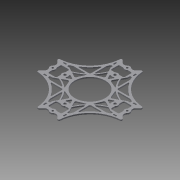
# Autodesk Inventor part: Middle Plate Under
Saved by Autodesk Inventor 2014 SP1 (Build 180222100, 222)
## iProperties
Created: 2014-07-28
Part Number: Middle Plate Under
Material: Generic
Document SubType Name: Modeling
Designer: Ryan
Density: 1 g/cm^3
Appearance: Default
Author: Ryan
Autodesk Inventor part; units mm, degrees
(part 1 of 2)
ref_plane "YZ Plane" through (0, 0, 0) normal (1, 0, 0) x (0, 1, 0)
ref_plane "XZ Plane" through (0, 0, 0) normal (0, 1, 0) x (-1, 0, 0)
ref_plane "XY Plane" through (0, 0, 0) normal (0, 0, 1) x (1, 0, 0)
sketch "Middle Plate Under" plane through (0, 0, 0) normal (0, 0, 1) x (1, 0, 0)
  arc A0 (50.1297, 0.9388) -> (0.939, 50.1217) centre (-2.2631, -2.2716) ccw
  arc A1 (50.1297, 0.9388) -> (51.1278, 0) centre (51.1278, 1) ccw
  arc A2 (0, 51.1198) -> (0.939, 50.1217) centre (1, 51.1198) ccw
  line L0 (5.9986, 74.9303) -> (5.9986, 74.6246)
  arc A3 (5.9986, 74.9303) -> (4.5341, 78.4659) centre (0.9986, 74.9303) ccw
  arc A4 (0.9376, 85.8703) -> (50.1218, 135.0623) centre (-2.3433, 138.3348) ccw
  arc A5 (0.9376, 85.8703) -> (0, 84.8722) centre (1, 84.8722) ccw
  arc A6 (51.1198, 136) -> (50.1218, 135.0623) centre (51.1198, 135) ccw
  arc A7 (135.0596, 50.1296) -> (85.8784, 0.9406) centre (138.1819, -2.1735) ccw
  arc A8 (84.8801, 0) -> (85.8784, 0.9406) centre (84.8801, 1) ccw
  arc A9 (135.0596, 50.1296) -> (136, 51.1278) centre (135, 51.1278) ccw
  arc A10 (85.8703, 135.0624) -> (135.0622, 85.8782) centre (138.334, 138.3425) ccw
  arc A11 (85.8703, 135.0624) -> (84.8722, 136) centre (84.8722, 135) ccw
  arc A12 (136, 84.8802) -> (135.0622, 85.8782) centre (135, 84.8802) ccw
  circle A13 centre (27.5084, 68) radius 2.1
  circle A14 centre (108.4916, 68) radius 2.1
  circle A15 centre (68, 108.4916) radius 2.1
  circle A16 centre (68, 27.5084) radius 2.1
  line L1 (14, 83) -> (9, 83)
  line L2 (14, 53) -> (9, 53)
  line L3 (9, 83) -> (9, 85.1)
  line L4 (9, 85.1) -> (14, 85.1)
  line L5 (14, 85.1) -> (14, 83)
  line L6 (14, 53) -> (14, 50.9)
  line L7 (14, 50.9) -> (9, 50.9)
  line L8 (9, 50.9) -> (9, 53)
  line L9 (122, 83) -> (127, 83)
  line L10 (122, 53) -> (127, 53)
  line L11 (127, 83) -> (127, 85.1)
  line L12 (127, 85.1) -> (122, 85.1)
  line L13 (122, 85.1) -> (122, 83)
  line L14 (122, 53) -> (122, 50.9)
  line L15 (122, 50.9) -> (127, 50.9)
  line L16 (127, 50.9) -> (127, 53)
  line L17 (53, 122) -> (53, 127)
  line L18 (83, 122) -> (83, 127)
  line L19 (53, 127) -> (50.9, 127)
  line L20 (50.9, 127) -> (50.9, 122)
  line L21 (50.9, 122) -> (53, 122)
  line L22 (83, 122) -> (85.1, 122)
  line L23 (85.1, 122) -> (85.1, 127)
  line L24 (85.1, 127) -> (83, 127)
  line L25 (53, 14) -> (53, 9)
  line L26 (83, 14) -> (83, 9)
  line L27 (53, 9) -> (50.9, 9)
  line L28 (50.9, 9) -> (50.9, 14)
  line L29 (50.9, 14) -> (53, 14)
  line L30 (83, 14) -> (85.1, 14)
  line L31 (85.1, 14) -> (85.1, 9)
  line L32 (85.1, 9) -> (83, 9)
  line L33 (12.5486, 78.8671) -> (22.185, 78.8671)
  arc A17 (12.5486, 78.8671) -> (10.6486, 76.9671) centre (12.5486, 76.9671) ccw
  line L34 (10.6486, 76.9671) -> (10.6486, 71.42)
  line L35 (24.085, 71.42) -> (24.085, 76.9671)
  arc A18 (24.085, 76.9671) -> (22.185, 78.8671) centre (22.185, 76.9671) ccw
  line L36 (12.5486, 57.1329) -> (22.185, 57.1329)
  arc A19 (10.6486, 59.0329) -> (12.5486, 57.1329) centre (12.5486, 59.0329) ccw
  line L37 (10.6486, 59.0329) -> (10.6486, 64.58)
  line L38 (24.085, 64.58) -> (24.085, 59.0329)
  arc A20 (22.185, 57.1329) -> (24.085, 59.0329) centre (22.185, 59.0329) ccw
  arc A21 (10.6486, 64.58) -> (10.6486, 71.42) centre (7.1826, 68) ccw
  arc A22 (24.085, 71.42) -> (24.085, 64.58) centre (27.505, 68) ccw
  line L39 (123.4514, 78.8671) -> (113.815, 78.8671)
  arc A23 (125.3514, 76.9671) -> (123.4514, 78.8671) centre (123.4514, 76.9671) ccw
  line L40 (125.3514, 76.9671) -> (125.3514, 71.42)
  line L41 (111.915, 71.42) -> (111.915, 76.9671)
  arc A24 (113.815, 78.8671) -> (111.915, 76.9671) centre (113.815, 76.9671) ccw
  line L42 (123.4514, 57.1329) -> (113.815, 57.1329)
  arc A25 (123.4514, 57.1329) -> (125.3514, 59.0329) centre (123.4514, 59.0329) ccw
  line L43 (125.3514, 59.0329) -> (125.3514, 64.58)
  line L44 (111.915, 64.58) -> (111.915, 59.0329)
  arc A26 (111.915, 59.0329) -> (113.815, 57.1329) centre (113.815, 59.0329) ccw
  arc A27 (125.3514, 71.42) -> (125.3514, 64.58) centre (128.8174, 68) ccw
  arc A28 (111.915, 64.58) -> (111.915, 71.42) centre (108.495, 68) ccw
  line L45 (57.1329, 123.4514) -> (57.1329, 113.815)
  arc A29 (59.0329, 125.3514) -> (57.1329, 123.4514) centre (59.0329, 123.4514) ccw
  line L46 (59.0329, 125.3514) -> (64.58, 125.3514)
  line L47 (64.58, 111.915) -> (59.0329, 111.915)
  arc A30 (57.1329, 113.815) -> (59.0329, 111.915) centre (59.0329, 113.815) ccw
  line L48 (78.8671, 123.4514) -> (78.8671, 113.815)
  arc A31 (78.8671, 123.4514) -> (76.9671, 125.3514) centre (76.9671, 123.4514) ccw
  line L49 (76.9671, 125.3514) -> (71.42, 125.3514)
  line L50 (71.42, 111.915) -> (76.9671, 111.915)
  arc A32 (76.9671, 111.915) -> (78.8671, 113.815) centre (76.9671, 113.815) ccw
  arc A33 (64.58, 125.3514) -> (71.42, 125.3514) centre (68, 128.8174) ccw
  arc A34 (71.42, 111.915) -> (64.58, 111.915) centre (68, 108.495) ccw
  line L51 (57.1329, 12.5486) -> (57.1329, 22.185)
  arc A35 (57.1329, 12.5486) -> (59.0329, 10.6486) centre (59.0329, 12.5486) ccw
  line L52 (59.0329, 10.6486) -> (64.58, 10.6486)
  line L53 (64.58, 24.085) -> (59.0329, 24.085)
  arc A36 (59.0329, 24.085) -> (57.1329, 22.185) centre (59.0329, 22.185) ccw
  line L54 (78.8671, 12.5486) -> (78.8671, 22.185)
  arc A37 (76.9671, 10.6486) -> (78.8671, 12.5486) centre (76.9671, 12.5486) ccw
  line L55 (76.9671, 10.6486) -> (71.42, 10.6486)
  line L56 (71.42, 24.085) -> (76.9671, 24.085)
  arc A38 (78.8671, 22.185) -> (76.9671, 24.085) centre (76.9671, 22.185) ccw
  arc A39 (71.42, 10.6486) -> (64.58, 10.6486) centre (68, 7.1826) ccw
  arc A40 (64.58, 24.085) -> (71.42, 24.085) centre (68, 27.505) ccw
  arc A41 (27.6448, 91.2527) -> (44.7476, 108.3555) centre (-2.445, 138.4453) ccw
  arc A42 (27.6448, 91.2527) -> (28.102, 89.6852) centre (28.102, 90.5356) ccw
  arc A43 (46.3151, 107.8983) -> (44.7476, 108.3555) centre (45.4647, 107.8983) ccw
  line L57 (40.2804, 87.1341) -> (22.5335, 87.1334)
  line L58 (44.1891, 89.6852) -> (28.102, 89.6852)
  line L59 (46.3151, 91.8112) -> (46.3151, 107.8983)
  arc A44 (44.1891, 89.6852) -> (46.3151, 91.8112) centre (44.1891, 91.8112) ccw
  arc A45 (27.1963, 78.4533) -> (28.6868, 78.3895) centre (28.007, 79.9485) ccw
  arc A46 (28.6868, 78.3895) -> (40.8045, 85.614) centre (6.3199, 129.6804) ccw
  line L60 (21.3459, 81.6253) -> (27.1963, 78.4533)
  line L61 (30.5408, 76.64) -> (37.2048, 73.0269)
  arc A47 (40.8045, 85.614) -> (40.2804, 87.1341) centre (40.2804, 86.2837) ccw
  arc A48 (91.2524, 108.3555) -> (108.3552, 91.2527) centre (138.445, 138.4453) ccw
  arc A49 (107.898, 89.6852) -> (108.3552, 91.2527) centre (107.898, 90.5356) ccw
  arc A50 (91.2524, 108.3555) -> (89.6849, 107.8983) centre (90.5353, 107.8983) ccw
  line L62 (91.8109, 89.6852) -> (107.898, 89.6852)
  line L63 (89.6849, 91.8112) -> (89.6849, 107.8983)
  arc A51 (89.6849, 91.8112) -> (91.8109, 89.6852) centre (91.8109, 91.8112) ccw
  arc A52 (108.3552, 44.7479) -> (91.2524, 27.6451) centre (138.445, -2.4447) ccw
  arc A53 (108.3552, 44.7479) -> (107.898, 46.3154) centre (107.898, 45.465) ccw
  arc A54 (89.6849, 28.1023) -> (91.2524, 27.6451) centre (90.5353, 28.1023) ccw
  line L64 (91.8109, 46.3154) -> (107.898, 46.3154)
  line L65 (89.6849, 44.1894) -> (89.6849, 28.1023)
  arc A55 (91.8109, 46.3154) -> (89.6849, 44.1894) centre (91.8109, 44.1894) ccw
  arc A56 (30.5752, 77.4043) -> (44.1261, 85.6969) centre (8.4389, 128.7951) ccw
  arc A57 (44.7901, 85.2067) -> (44.1261, 85.6969) centre (44.3973, 85.3694) ccw
  arc A58 (30.5752, 77.4043) -> (30.5408, 76.64) centre (30.7434, 77.0138) ccw
  line L66 (44.7901, 85.2067) -> (40.1822, 74.0823)
  arc A59 (37.2048, 73.0269) -> (40.1822, 74.0823) centre (38.2181, 74.8959) ccw
  line L67 (30.5408, 59.3606) -> (37.2048, 62.9737)
  arc A60 (40.1822, 61.9183) -> (37.2048, 62.9737) centre (38.2181, 61.1047) ccw
  arc A61 (44.1261, 50.3037) -> (30.5752, 58.5963) centre (8.4389, 7.2055) ccw
  arc A62 (44.1261, 50.3037) -> (44.7901, 50.7939) centre (44.3973, 50.6312) ccw
  arc A63 (30.5408, 59.3606) -> (30.5752, 58.5963) centre (30.7434, 58.9868) ccw
  line L68 (44.7901, 50.7939) -> (40.1822, 61.9183)
  line L69 (105.4592, 76.64) -> (98.7952, 73.0269)
  arc A64 (91.8739, 85.6969) -> (105.4248, 77.4043) centre (127.5611, 128.7951) ccw
  arc A65 (91.8739, 85.6969) -> (91.2099, 85.2067) centre (91.6027, 85.3694) ccw
  arc A66 (105.4592, 76.64) -> (105.4248, 77.4043) centre (105.2566, 77.0138) ccw
  line L70 (91.2099, 85.2067) -> (95.8178, 74.0823)
  arc A67 (95.8178, 74.0823) -> (98.7952, 73.0269) centre (97.7819, 74.8959) ccw
  line L71 (105.4592, 59.3606) -> (98.7952, 62.9737)
  arc A68 (98.7952, 62.9737) -> (95.8178, 61.9183) centre (97.7819, 61.1047) ccw
  arc A69 (105.4248, 58.5963) -> (91.8739, 50.3037) centre (127.5611, 7.2055) ccw
  arc A70 (91.2099, 50.7939) -> (91.8739, 50.3037) centre (91.6027, 50.6312) ccw
  arc A71 (105.4248, 58.5963) -> (105.4592, 59.3606) centre (105.2566, 58.9868) ccw
  line L72 (91.2099, 50.7939) -> (95.8178, 61.9183)
  line L73 (59.3603, 105.4595) -> (62.9734, 98.7955)
  arc A72 (61.918, 95.8181) -> (62.9734, 98.7955) centre (61.1044, 97.7822) ccw
  arc A73 (50.3034, 91.8742) -> (58.596, 105.4251) centre (7.2052, 127.5614) ccw
  arc A74 (50.3034, 91.8742) -> (50.7936, 91.2102) centre (50.6309, 91.603) ccw
  arc A75 (59.3603, 105.4595) -> (58.596, 105.4251) centre (58.9865, 105.2569) ccw
  line L74 (50.7936, 91.2102) -> (61.918, 95.8181)
  line L75 (76.6397, 105.4595) -> (73.0266, 98.7955)
  arc A76 (73.0266, 98.7955) -> (74.082, 95.8181) centre (74.8956, 97.7822) ccw
  arc A77 (77.404, 105.4251) -> (85.6966, 91.8742) centre (128.7948, 127.5614) ccw
  arc A78 (85.2064, 91.2102) -> (85.6966, 91.8742) centre (85.3691, 91.603) ccw
  arc A79 (77.404, 105.4251) -> (76.6397, 105.4595) centre (77.0135, 105.2569) ccw
  line L76 (85.2064, 91.2102) -> (74.082, 95.8181)
  line L77 (59.3603, 30.5411) -> (62.9734, 37.2051)
  arc A80 (62.9734, 37.2051) -> (61.918, 40.1825) centre (61.1044, 38.2184) ccw
  arc A81 (58.596, 30.5755) -> (50.3034, 44.1264) centre (7.2052, 8.4392) ccw
  arc A82 (50.7936, 44.7904) -> (50.3034, 44.1264) centre (50.6309, 44.3976) ccw
  arc A83 (58.596, 30.5755) -> (59.3603, 30.5411) centre (58.9865, 30.7437) ccw
  line L78 (50.7936, 44.7904) -> (61.918, 40.1825)
  line L79 (76.6397, 30.5411) -> (73.0266, 37.2051)
  arc A84 (85.6966, 44.1264) -> (77.404, 30.5755) centre (128.7948, 8.4392) ccw
  arc A85 (85.6966, 44.1264) -> (85.2064, 44.7904) centre (85.3691, 44.3976) ccw
  arc A86 (76.6397, 30.5411) -> (77.404, 30.5755) centre (77.0135, 30.7437) ccw
  line L80 (85.2064, 44.7904) -> (74.082, 40.1825)
  arc A87 (74.082, 40.1825) -> (73.0266, 37.2051) centre (74.8956, 38.2184) ccw
  circle A88 centre (68, 68) radius 24.5933
  arc A89 (44.7476, 27.6451) -> (27.6448, 44.7479) centre (-2.445, -2.4447) ccw
  arc A90 (44.7476, 27.6451) -> (46.3151, 28.1023) centre (45.4647, 28.1023) ccw
  arc A91 (28.102, 46.3154) -> (27.6448, 44.7479) centre (28.102, 45.465) ccw
  line L81 (46.3151, 44.1894) -> (46.3151, 28.1023)
  line L82 (44.1891, 46.3154) -> (28.102, 46.3154)
  arc A92 (46.3151, 44.1894) -> (44.1891, 46.3154) centre (44.1891, 44.1894) ccw
  line L83 (64.2924, 102.9057) -> (67.1209, 97.6888)
  arc A93 (67.1209, 97.6888) -> (68.8791, 97.6888) centre (68, 98.1654) ccw
  line L84 (71.7076, 102.9057) -> (68.8791, 97.6888)
  arc A94 (65.6558, 104.2572) -> (70.3442, 104.2572) centre (68, 108.4916) ccw
  arc A95 (65.6558, 104.2572) -> (64.2924, 102.9057) centre (65.1715, 103.3823) ccw
  arc A96 (71.7076, 102.9057) -> (70.3442, 104.2572) centre (70.8285, 103.3823) ccw
  line L85 (64.2924, 33.0943) -> (67.1209, 38.3112)
  arc A97 (68.8791, 38.3112) -> (67.1209, 38.3112) centre (68, 37.8346) ccw
  line L86 (71.7076, 33.0943) -> (68.8791, 38.3112)
  arc A98 (70.3442, 31.7428) -> (65.6558, 31.7428) centre (68, 27.5084) ccw
  arc A99 (64.2924, 33.0943) -> (65.6558, 31.7428) centre (65.1715, 32.6177) ccw
  arc A100 (70.3442, 31.7428) -> (71.7076, 33.0943) centre (70.8285, 32.6177) ccw
  line L87 (33.0946, 71.7079) -> (38.3115, 68.8794)
  arc A101 (38.3115, 67.1212) -> (38.3115, 68.8794) centre (37.8349, 68.0003) ccw
  line L88 (33.0946, 64.2927) -> (38.3115, 67.1212)
  arc A102 (31.7431, 65.6561) -> (31.7431, 70.3445) centre (27.5087, 68.0003) ccw
  arc A103 (33.0946, 71.7079) -> (31.7431, 70.3445) centre (32.618, 70.8288) ccw
  arc A104 (31.7431, 65.6561) -> (33.0946, 64.2927) centre (32.618, 65.1718) ccw
  line L89 (102.906, 71.7079) -> (97.6891, 68.8794)
  arc A105 (97.6891, 68.8794) -> (97.6891, 67.1212) centre (98.1657, 68.0003) ccw
  line L90 (102.906, 64.2927) -> (97.6891, 67.1212)
  arc A106 (104.2575, 70.3445) -> (104.2575, 65.6561) centre (108.4919, 68.0003) ccw
  arc A107 (104.2575, 70.3445) -> (102.906, 71.7079) centre (103.3826, 70.8288) ccw
  arc A108 (102.906, 64.2927) -> (104.2575, 65.6561) centre (103.3826, 65.1718) ccw
  circle A109 centre (7.7484, 68) radius 1.6
  circle A110 centre (128.2516, 68) radius 1.6
  circle A111 centre (68, 128.2516) radius 1.6
  circle A112 centre (68, 7.7484) radius 1.6
  arc A113 (4.7048, 71.2684) -> (4.7048, 64.7316) centre (8.3141, 68) ccw
  arc A114 (5.9986, 61.3754) -> (4.7048, 64.7316) centre (0.9986, 61.3754) ccw
  arc A115 (4.7048, 71.2684) -> (5.9986, 74.6246) centre (0.9986, 74.6246) ccw
  arc A116 (131.2952, 64.7316) -> (131.2952, 71.2684) centre (127.6859, 68) ccw
  arc A117 (131.2952, 64.7316) -> (130.0014, 61.3754) centre (135.0014, 61.3754) ccw
  arc A118 (130.0014, 74.6246) -> (131.2952, 71.2684) centre (135.0014, 74.6246) ccw
  arc A119 (71.2684, 131.2952) -> (64.7316, 131.2952) centre (68, 127.6859) ccw
  arc A120 (71.2684, 131.2952) -> (74.6246, 130.0014) centre (74.6246, 135.0014) ccw
  arc A121 (61.3754, 130.0014) -> (64.7316, 131.2952) centre (61.3754, 135.0014) ccw
  arc A122 (64.7316, 4.7048) -> (71.2684, 4.7048) centre (68, 8.3141) ccw
  arc A123 (64.7316, 4.7048) -> (61.3754, 5.9986) centre (61.3754, 0.9986) ccw
  arc A124 (74.6246, 5.9986) -> (71.2684, 4.7048) centre (74.6246, 0.9986) ccw
  line L91 (17, 83.6623) -> (17, 82.8671)
  arc A125 (18.2965, 85.5345) -> (21.7007, 86.9517) centre (-0.1983, 134.7566) ccw
  arc A126 (18.2965, 85.5345) -> (17, 83.6623) centre (19, 83.6623) ccw
  arc A127 (22.5335, 87.1334) -> (21.7007, 86.9517) centre (22.5336, 85.1334) ccw
  line L92 (18, 81.8671) -> (20.3926, 81.8671)
  arc A128 (17, 82.8671) -> (18, 81.8671) centre (18, 82.8671) ccw
  arc A129 (21.3459, 81.6253) -> (20.3926, 81.8671) centre (20.3926, 79.8671) ccw
  line L93 (40.2804, 48.8659) -> (22.5335, 48.8666)
  arc A130 (28.6868, 57.6105) -> (27.1963, 57.5467) centre (28.007, 56.0515) ccw
  arc A131 (40.8045, 50.386) -> (28.6868, 57.6105) centre (6.3199, 6.3196) ccw
  line L94 (21.3459, 54.3747) -> (27.1963, 57.5467)
  arc A132 (40.2804, 48.8659) -> (40.8045, 50.386) centre (40.2804, 49.7163) ccw
  line L95 (17, 52.3377) -> (17, 53.1329)
  arc A133 (21.7007, 49.0483) -> (18.2965, 50.4655) centre (-0.1983, 1.2434) ccw
  arc A134 (17, 52.3377) -> (18.2965, 50.4655) centre (19, 52.3377) ccw
  arc A135 (21.7007, 49.0483) -> (22.5335, 48.8666) centre (22.5336, 50.8666) ccw
  line L96 (18, 54.1329) -> (20.3926, 54.1329)
  arc A136 (18, 54.1329) -> (17, 53.1329) centre (18, 53.1329) ccw
  arc A137 (20.3926, 54.1329) -> (21.3459, 54.3747) centre (20.3926, 56.1329) ccw
  line L97 (95.7196, 87.1341) -> (113.4665, 87.1334)
  arc A138 (107.3132, 78.3895) -> (108.8037, 78.4533) centre (107.993, 79.9485) ccw
  arc A139 (95.1955, 85.614) -> (107.3132, 78.3895) centre (129.6801, 129.6804) ccw
  line L98 (114.6541, 81.6253) -> (108.8037, 78.4533)
  arc A140 (95.7196, 87.1341) -> (95.1955, 85.614) centre (95.7196, 86.2837) ccw
  line L99 (119, 83.6623) -> (119, 82.8671)
  arc A141 (114.2993, 86.9517) -> (117.7035, 85.5345) centre (136.1983, 134.7566) ccw
  arc A142 (119, 83.6623) -> (117.7035, 85.5345) centre (117, 83.6623) ccw
  arc A143 (114.2993, 86.9517) -> (113.4665, 87.1334) centre (113.4664, 85.1334) ccw
  line L100 (118, 81.8671) -> (115.6074, 81.8671)
  arc A144 (118, 81.8671) -> (119, 82.8671) centre (118, 82.8671) ccw
  arc A145 (115.6074, 81.8671) -> (114.6541, 81.6253) centre (115.6074, 79.8671) ccw
  line L101 (95.7196, 48.8659) -> (113.4665, 48.8666)
  arc A146 (108.8037, 57.5467) -> (107.3132, 57.6105) centre (107.993, 56.0515) ccw
  arc A147 (107.3132, 57.6105) -> (95.1955, 50.386) centre (129.6801, 6.3196) ccw
  line L102 (114.6541, 54.3747) -> (108.8037, 57.5467)
  arc A148 (95.1955, 50.386) -> (95.7196, 48.8659) centre (95.7196, 49.7163) ccw
  line L103 (119, 52.3377) -> (119, 53.1329)
  arc A149 (117.7035, 50.4655) -> (114.2993, 49.0483) centre (136.1983, 1.2434) ccw
  arc A150 (117.7035, 50.4655) -> (119, 52.3377) centre (117, 52.3377) ccw
  arc A151 (113.4665, 48.8666) -> (114.2993, 49.0483) centre (113.4664, 50.8666) ccw
  line L104 (118, 54.1329) -> (115.6074, 54.1329)
  arc A152 (119, 53.1329) -> (118, 54.1329) centre (118, 53.1329) ccw
  arc A153 (114.6541, 54.3747) -> (115.6074, 54.1329) centre (115.6074, 56.1329) ccw
  line L105 (48.8662, 40.2807) -> (48.8669, 22.5339)
  arc A154 (57.547, 27.1966) -> (57.6108, 28.6871) centre (56.0518, 28.0073) ccw
  arc A155 (57.6108, 28.6871) -> (50.3863, 40.8048) centre (6.3199, 6.3202) ccw
  line L106 (54.375, 21.3462) -> (57.547, 27.1966)
  arc A156 (50.3863, 40.8048) -> (48.8662, 40.2807) centre (49.7166, 40.2807) ccw
  line L107 (52.338, 17.0003) -> (53.1332, 17.0003)
  arc A157 (50.4658, 18.2968) -> (49.0486, 21.701) centre (1.2437, -0.198) ccw
  arc A158 (50.4658, 18.2968) -> (52.338, 17.0003) centre (52.338, 19.0003) ccw
  arc A159 (48.8669, 22.5339) -> (49.0486, 21.701) centre (50.8669, 22.5339) ccw
  line L108 (54.1332, 18.0003) -> (54.1332, 20.3929)
  arc A160 (53.1332, 17.0003) -> (54.1332, 18.0003) centre (53.1332, 18.0003) ccw
  arc A161 (54.375, 21.3462) -> (54.1332, 20.3929) centre (56.1332, 20.3929) ccw
  line L109 (87.1344, 40.2807) -> (87.1337, 22.5339)
  arc A162 (78.3898, 28.6871) -> (78.4536, 27.1966) centre (79.9488, 28.0073) ccw
  arc A163 (85.6143, 40.8048) -> (78.3898, 28.6871) centre (129.6807, 6.3202) ccw
  line L110 (81.6256, 21.3462) -> (78.4536, 27.1966)
  arc A164 (87.1344, 40.2807) -> (85.6143, 40.8048) centre (86.284, 40.2807) ccw
  line L111 (83.6626, 17.0003) -> (82.8674, 17.0003)
  arc A165 (86.952, 21.701) -> (85.5348, 18.2968) centre (134.7569, -0.198) ccw
  arc A166 (83.6626, 17.0003) -> (85.5348, 18.2968) centre (83.6626, 19.0003) ccw
  line L112 (87.1344, 95.7199) -> (87.1337, 113.4668)
  arc A167 (86.952, 21.701) -> (87.1337, 22.5339) centre (85.1337, 22.5339) ccw
  line L113 (81.8674, 18.0003) -> (81.8674, 20.3929)
  arc A168 (81.8674, 18.0003) -> (82.8674, 17.0003) centre (82.8674, 18.0003) ccw
  arc A169 (81.8674, 20.3929) -> (81.6256, 21.3462) centre (79.8674, 20.3929) ccw
  line L114 (48.8662, 95.7199) -> (48.8669, 113.4668)
  arc A170 (57.6108, 107.3135) -> (57.547, 108.804) centre (56.0518, 107.9933) ccw
  arc A171 (50.3863, 95.1958) -> (57.6108, 107.3135) centre (6.3199, 129.6804) ccw
  line L115 (54.375, 114.6544) -> (57.547, 108.804)
  arc A172 (48.8662, 95.7199) -> (50.3863, 95.1958) centre (49.7166, 95.7199) ccw
  line L116 (52.338, 119.0003) -> (53.1332, 119.0003)
  arc A173 (49.0486, 114.2996) -> (50.4658, 117.7038) centre (1.2437, 136.1986) ccw
  arc A174 (52.338, 119.0003) -> (50.4658, 117.7038) centre (52.338, 117.0003) ccw
  arc A175 (49.0486, 114.2996) -> (48.8669, 113.4668) centre (50.8669, 113.4667) ccw
  line L117 (54.1332, 118.0003) -> (54.1332, 115.6077)
  arc A176 (54.1332, 118.0003) -> (53.1332, 119.0003) centre (53.1332, 118.0003) ccw
  arc A177 (54.1332, 115.6077) -> (54.375, 114.6544) centre (56.1332, 115.6077) ccw
  arc A178 (78.4536, 108.804) -> (78.3898, 107.3135) centre (79.9488, 107.9933) ccw
  arc A179 (85.6143, 95.1958) -> (87.1344, 95.7199) centre (86.284, 95.7199) ccw
  arc A180 (78.3898, 107.3135) -> (85.6143, 95.1958) centre (129.6807, 129.6804) ccw
  line L118 (81.6256, 114.6544) -> (78.4536, 108.804)
  line L119 (83.6626, 119.0003) -> (82.8674, 119.0003)
  arc A181 (85.5348, 117.7038) -> (86.952, 114.2996) centre (134.7569, 136.1986) ccw
  arc A182 (85.5348, 117.7038) -> (83.6626, 119.0003) centre (83.6626, 117.0003) ccw
  arc A183 (87.1337, 113.4668) -> (86.952, 114.2996) centre (85.1337, 113.4667) ccw
  line L120 (81.8674, 118.0003) -> (81.8674, 115.6077)
  arc A184 (82.8674, 119.0003) -> (81.8674, 118.0003) centre (82.8674, 118.0003) ccw
  arc A185 (81.6256, 114.6544) -> (81.8674, 115.6077) centre (79.8674, 115.6077) ccw
  line L121 (0, 83.4142) -> (0, 84.8722)
  arc A186 (0, 83.4142) -> (0.2929, 82.7071) centre (1, 83.4142) ccw
  line L122 (4.5341, 78.4659) -> (0.2929, 82.7071)
  line L123 (5.9986, 61.0697) -> (5.9986, 61.3754)
  line L124 (0, 52.5858) -> (0, 51.1198)
  line L125 (4.5341, 57.5341) -> (0.2929, 53.2929)
  arc A187 (4.5341, 57.5341) -> (5.9986, 61.0697) centre (0.9986, 61.0697) ccw
  arc A188 (0.2929, 53.2929) -> (0, 52.5858) centre (1, 52.5858) ccw
  line L126 (61.0697, 5.9986) -> (61.3754, 5.9986)
  line L127 (52.5858, 0) -> (51.1278, 0)
  line L128 (57.5341, 4.5341) -> (53.2929, 0.2929)
  arc A189 (61.0697, 5.9986) -> (57.5341, 4.5341) centre (61.0697, 0.9986) ccw
  arc A190 (52.5858, 0) -> (53.2929, 0.2929) centre (52.5858, 1) ccw
  line L129 (74.9303, 5.9986) -> (74.6246, 5.9986)
  arc A191 (78.4659, 4.5341) -> (74.9303, 5.9986) centre (74.9303, 0.9986) ccw
  line L130 (83.4142, 0) -> (84.8801, 0)
  arc A192 (82.7071, 0.2929) -> (83.4142, 0) centre (83.4142, 1) ccw
  line L131 (78.4659, 4.5341) -> (82.7071, 0.2929)
  line L132 (130.0014, 61.0697) -> (130.0014, 61.3754)
  line L133 (136, 52.5858) -> (136, 51.1278)
  arc A193 (136, 52.5858) -> (135.7071, 53.2929) centre (135, 52.5858) ccw
  line L134 (131.4659, 57.5341) -> (135.7071, 53.2929)
  arc A194 (130.0014, 61.0697) -> (131.4659, 57.5341) centre (135.0014, 61.0697) ccw
  line L135 (130.0014, 74.9303) -> (130.0014, 74.6246)
  arc A195 (131.4659, 78.4659) -> (130.0014, 74.9303) centre (135.0014, 74.9303) ccw
  line L136 (136, 83.4142) -> (136, 84.8802)
  arc A196 (135.7071, 82.7071) -> (136, 83.4142) centre (135, 83.4142) ccw
  line L137 (131.4659, 78.4659) -> (135.7071, 82.7071)
  line L138 (74.9303, 130.0014) -> (74.6246, 130.0014)
  line L139 (83.4142, 136) -> (84.8722, 136)
  arc A197 (83.4142, 136) -> (82.7071, 135.7071) centre (83.4142, 135) ccw
  line L140 (78.4659, 131.4659) -> (82.7071, 135.7071)
  arc A198 (74.9303, 130.0014) -> (78.4659, 131.4659) centre (74.9303, 135.0014) ccw
  line L141 (61.0697, 130.0014) -> (61.3754, 130.0014)
  arc A199 (57.5341, 131.4659) -> (61.0697, 130.0014) centre (61.0697, 135.0014) ccw
  line L142 (52.5858, 136) -> (51.1198, 136)
  arc A200 (53.2929, 135.7071) -> (52.5858, 136) centre (52.5858, 135) ccw
  line L143 (57.5341, 131.4659) -> (53.2929, 135.7071)
  point P0 (68, 68.0003)
sketch "Sketch1" plane through (0, 0, 0) normal (0, 1, 0) x (-1, 0, 0)
  circle A0 centre (68, 68) radius 24.5933
  circle A1 centre (108.495, 68) radius 2.1034
  circle A2 centre (68, 27.505) radius 2.1
  circle A3 centre (27.505, 68) radius 2.1034
  circle A4 centre (68, 108.495) radius 2.1
  circle A5 centre (68, 128.2516) radius 1.6
  circle A6 centre (128.2516, 68) radius 1.6
  circle A7 centre (68, 7.7484) radius 1.6
  circle A8 centre (7.7484, 68) radius 1.6
  line L0 (9, 53) -> (14, 53)
  line L1 (14, 53) -> (14, 50.9)
  line L2 (14, 50.9) -> (9, 50.9)
  line L3 (9, 50.9) -> (9, 53)
  line L4 (9, 85.1) -> (14, 85.1)
  line L5 (14, 85.1) -> (14, 83)
  line L6 (14, 83) -> (9, 83)
  line L7 (9, 83) -> (9, 85.1)
  line L8 (50.9, 127) -> (53, 127)
  line L9 (53, 127) -> (53, 122)
  line L10 (53, 122) -> (50.9, 122)
  line L11 (50.9, 122) -> (50.9, 127)
  line L12 (83, 127) -> (85.1, 127)
  line L13 (85.1, 127) -> (85.1, 122)
  line L14 (85.1, 122) -> (83, 122)
  line L15 (83, 122) -> (83, 127)
  line L16 (122, 85.1) -> (127, 85.1)
  line L17 (127, 85.1) -> (127, 83)
  line L18 (127, 83) -> (122, 83)
  line L19 (122, 83) -> (122, 85.1)
  line L20 (127, 53) -> (122, 53)
  line L21 (122, 53) -> (122, 50.9)
  line L22 (122, 50.9) -> (127, 50.9)
  line L23 (127, 50.9) -> (127, 53)
  line L24 (50.9, 14) -> (53, 14)
  line L25 (53, 14) -> (53, 9)
  line L26 (53, 9) -> (50.9, 9)
  line L27 (50.9, 9) -> (50.9, 14)
  line L28 (83, 14) -> (85.1, 14)
  line L29 (85.1, 14) -> (85.1, 9)
  line L30 (85.1, 9) -> (83, 9)
  line L31 (83, 9) -> (83, 14)
  arc A9 (0.9376, 85.8703) -> (0, 84.8722) centre (1, 84.8722) ccw
  arc A10 (0, 83.4142) -> (0.2929, 82.7071) centre (1, 83.4142) ccw
  arc A11 (51.1198, 136) -> (50.1218, 135.0623) centre (51.1198, 135) ccw
  arc A12 (53.2929, 135.7071) -> (52.5858, 136) centre (52.5858, 135) ccw
  arc A13 (83.4142, 136) -> (82.7071, 135.7071) centre (83.4142, 135) ccw
  arc A14 (85.8703, 135.0624) -> (84.8722, 136) centre (84.8722, 135) ccw
  arc A15 (136, 84.8802) -> (135.0622, 85.8782) centre (135, 84.8802) ccw
  arc A16 (135.7071, 82.7071) -> (136, 83.4142) centre (135, 83.4142) ccw
  arc A17 (135.0596, 50.1296) -> (136, 51.1278) centre (135, 51.1278) ccw
  arc A18 (136, 52.5858) -> (135.7071, 53.2929) centre (135, 52.5858) ccw
  arc A19 (84.8801, 0) -> (85.8784, 0.9406) centre (84.8801, 1) ccw
  arc A20 (82.7071, 0.2929) -> (83.4142, 0) centre (83.4142, 1) ccw
  arc A21 (0, 51.1198) -> (0.939, 50.1217) centre (1, 51.1198) ccw
  arc A22 (0.2929, 53.2929) -> (0, 52.5858) centre (1, 52.5858) ccw
  arc A23 (135.0596, 50.1296) -> (85.8784, 0.9406) centre (138.1819, -2.1735) ccw
  arc A24 (50.1297, 0.9388) -> (0.939, 50.1217) centre (-2.2631, -2.2716) ccw
  arc A25 (0.9376, 85.8703) -> (50.1218, 135.0623) centre (-2.3433, 138.3348) ccw
  arc A26 (85.8703, 135.0624) -> (135.0622, 85.8782) centre (138.334, 138.3425) ccw
  line L32 (51.1198, 136) -> (52.5858, 136)
  line L33 (53.2929, 135.7071) -> (57.5341, 131.4659)
  line L34 (78.4659, 131.4659) -> (82.7071, 135.7071)
  line L35 (83.4142, 136) -> (84.8722, 136)
  line L36 (136, 51.1278) -> (136, 52.5858)
  line L37 (136, 84.8802) -> (136, 83.4142)
  arc A27 (71.2684, 131.2952) -> (64.7316, 131.2952) centre (68, 127.6859) ccw
  arc A28 (71.2684, 131.2952) -> (74.6246, 130.0014) centre (74.6246, 135.0014) ccw
  arc A29 (74.9303, 130.0014) -> (78.4659, 131.4659) centre (74.9303, 135.0014) ccw
  line L38 (74.9303, 130.0014) -> (74.6246, 130.0014)
  arc A30 (61.3754, 130.0014) -> (64.7316, 131.2952) centre (61.3754, 135.0014) ccw
  arc A31 (57.5341, 131.4659) -> (61.0697, 130.0014) centre (61.0697, 135.0014) ccw
  line L39 (61.0697, 130.0014) -> (61.3754, 130.0014)
  arc A32 (131.4659, 78.4659) -> (130.0014, 74.9303) centre (135.0014, 74.9303) ccw
  arc A33 (130.0014, 74.6246) -> (131.2952, 71.2684) centre (135.0014, 74.6246) ccw
  line L40 (130.0014, 74.6246) -> (130.0014, 74.9303)
  arc A34 (130.0014, 61.0697) -> (131.4659, 57.5341) centre (135.0014, 61.0697) ccw
  arc A35 (131.2952, 64.7316) -> (130.0014, 61.3754) centre (135.0014, 61.3754) ccw
  line L41 (130.0014, 61.3754) -> (130.0014, 61.0697)
  arc A36 (131.2952, 64.7316) -> (131.2952, 71.2684) centre (127.6859, 68) ccw
  line L42 (131.4659, 57.5341) -> (135.7071, 53.2929)
  line L43 (131.4659, 78.4659) -> (135.7071, 82.7071)
  line L44 (84.8801, 0) -> (83.4142, 0)
  arc A37 (61.0697, 5.9986) -> (57.5341, 4.5341) centre (61.0697, 0.9986) ccw
  arc A38 (78.4659, 4.5341) -> (74.9303, 5.9986) centre (74.9303, 0.9986) ccw
  arc A39 (74.6246, 5.9986) -> (71.2684, 4.7048) centre (74.6246, 0.9986) ccw
  line L45 (74.6246, 5.9986) -> (74.9303, 5.9986)
  line L46 (78.4659, 4.5341) -> (82.7071, 0.2929)
  arc A40 (64.7316, 4.7048) -> (71.2684, 4.7048) centre (68, 8.3141) ccw
  line L47 (0, 51.1198) -> (0, 52.5858)
  line L48 (0, 83.4142) -> (0, 84.8722)
  arc A41 (5.9986, 61.3754) -> (4.7048, 64.7316) centre (0.9986, 61.3754) ccw
  arc A42 (4.5341, 57.5341) -> (5.9986, 61.0697) centre (0.9986, 61.0697) ccw
  line L49 (0.2929, 53.2929) -> (4.5341, 57.5341)
  line L50 (5.9986, 61.0697) -> (5.9986, 61.3754)
  arc A43 (4.7048, 71.2684) -> (4.7048, 64.7316) centre (8.3141, 68) ccw
  arc A44 (10.6486, 64.58) -> (10.6486, 71.42) centre (7.1826, 68) ccw
  arc A45 (24.085, 71.42) -> (24.085, 64.58) centre (27.505, 68) ccw
  arc A46 (31.7538, 65.6751) -> (31.7431, 70.3445) centre (27.505, 68) ccw
  arc A47 (22.185, 57.1329) -> (24.085, 59.0329) centre (22.185, 59.0329) ccw
  arc A48 (10.6486, 59.0329) -> (12.5486, 57.1329) centre (12.5486, 59.0329) ccw
  arc A49 (12.5486, 78.8671) -> (10.6486, 76.9671) centre (12.5486, 76.9671) ccw
  arc A50 (24.085, 76.9671) -> (22.185, 78.8671) centre (22.185, 76.9671) ccw
  line L51 (24.085, 76.9671) -> (24.085, 71.42)
  line L52 (10.6486, 71.42) -> (10.6486, 76.9671)
  line L53 (12.5486, 78.8671) -> (22.185, 78.8671)
  line L54 (24.085, 64.58) -> (24.085, 59.0329)
  line L55 (22.185, 57.1329) -> (12.5486, 57.1329)
  line L56 (10.6486, 59.0329) -> (10.6486, 64.58)
  arc A51 (31.7538, 65.6751) -> (33.0946, 64.2927) centre (32.618, 65.1718) ccw
  arc A52 (38.3115, 67.1212) -> (38.3115, 68.8794) centre (37.8349, 68.0003) ccw
  arc A53 (33.0946, 71.7079) -> (31.7431, 70.3445) centre (32.618, 70.8288) ccw
  line L57 (33.0946, 71.7079) -> (38.3115, 68.8794)
  line L58 (38.3115, 67.1212) -> (33.0946, 64.2927)
  arc A54 (17, 82.8671) -> (18, 81.8671) centre (18, 82.8671) ccw
  arc A55 (18.2965, 85.5345) -> (17, 83.6623) centre (19, 83.6623) ccw
  arc A56 (22.5335, 87.1334) -> (21.7007, 86.9517) centre (22.5336, 85.1334) ccw
  arc A57 (27.1963, 78.4533) -> (28.6868, 78.3895) centre (28.007, 79.9485) ccw
  arc A58 (40.8045, 85.614) -> (40.2804, 87.1341) centre (40.2804, 86.2837) ccw
  arc A59 (28.6868, 78.3895) -> (40.8045, 85.614) centre (6.3199, 129.6804) ccw
  line L59 (22.5335, 87.1334) -> (40.2804, 87.1341)
  line L60 (27.1963, 78.4533) -> (21.3459, 81.6253)
  line L61 (17, 82.8671) -> (17, 83.6623)
  arc A60 (18.2965, 85.5345) -> (21.7007, 86.9517) centre (-0.1983, 134.7566) ccw
  arc A61 (30.5752, 77.4043) -> (30.5408, 76.64) centre (30.7434, 77.0138) ccw
  arc A62 (37.2048, 73.0269) -> (40.1822, 74.0823) centre (38.2181, 74.8959) ccw
  arc A63 (44.7901, 85.2067) -> (44.1261, 85.6969) centre (44.3973, 85.3694) ccw
  arc A64 (30.5752, 77.4043) -> (44.1261, 85.6969) centre (8.4389, 128.7951) ccw
  line L62 (37.2048, 73.0269) -> (30.5408, 76.64)
  line L63 (40.1822, 74.0823) -> (44.7901, 85.2067)
  arc A65 (20.3926, 54.1329) -> (21.3459, 54.3747) centre (20.3926, 56.1329) ccw
  arc A66 (18, 54.1329) -> (17, 53.1329) centre (18, 53.1329) ccw
  arc A67 (17, 52.3377) -> (18.2965, 50.4655) centre (19, 52.3377) ccw
  arc A68 (21.7007, 49.0483) -> (22.5335, 48.8666) centre (22.5336, 50.8666) ccw
  arc A69 (40.2804, 48.8659) -> (40.8045, 50.386) centre (40.2804, 49.7163) ccw
  arc A70 (21.7007, 49.0483) -> (18.2965, 50.4655) centre (-0.1983, 1.2434) ccw
  line L64 (17, 52.3377) -> (17, 53.1329)
  line L65 (18, 54.1329) -> (20.3926, 54.1329)
  line L66 (22.5335, 48.8666) -> (40.2804, 48.8659)
  arc A71 (40.1822, 61.9183) -> (37.2048, 62.9737) centre (38.2181, 61.1047) ccw
  arc A72 (44.1261, 50.3037) -> (44.7901, 50.7939) centre (44.3973, 50.6312) ccw
  line L67 (40.1822, 61.9183) -> (44.7901, 50.7939)
  arc A73 (44.1261, 50.3037) -> (30.5752, 58.5963) centre (8.4389, 7.2055) ccw
  arc A74 (44.1891, 89.6852) -> (46.3151, 91.8112) centre (44.1891, 91.8112) ccw
  arc A75 (27.6448, 91.2527) -> (28.102, 89.6852) centre (28.102, 90.5356) ccw
  arc A76 (46.3151, 107.8983) -> (44.7476, 108.3555) centre (45.4647, 107.8983) ccw
  arc A77 (27.6448, 91.2527) -> (44.7476, 108.3555) centre (-2.445, 138.4453) ccw
  line L68 (46.3151, 107.8983) -> (46.3151, 91.8112)
  line L69 (44.1891, 89.6852) -> (28.102, 89.6852)
  arc A78 (46.3151, 44.1894) -> (44.1891, 46.3154) centre (44.1891, 44.1894) ccw
  arc A79 (44.7476, 27.6451) -> (46.3151, 28.1023) centre (45.4647, 28.1023) ccw
  arc A80 (28.102, 46.3154) -> (27.6448, 44.7479) centre (28.102, 45.465) ccw
  line L70 (28.102, 46.3154) -> (44.1891, 46.3154)
  line L71 (46.3151, 44.1894) -> (46.3151, 28.1023)
  arc A81 (44.7476, 27.6451) -> (27.6448, 44.7479) centre (-2.445, -2.4447) ccw
  arc A82 (71.42, 10.6486) -> (64.58, 10.6486) centre (68, 7.1826) ccw
  arc A83 (64.58, 24.085) -> (71.42, 24.085) centre (68, 27.505) ccw
  arc A84 (59.0329, 24.085) -> (57.1329, 22.185) centre (59.0329, 22.185) ccw
  arc A85 (78.8671, 22.185) -> (76.9671, 24.085) centre (76.9671, 22.185) ccw
  arc A86 (76.9671, 10.6486) -> (78.8671, 12.5486) centre (76.9671, 12.5486) ccw
  arc A87 (57.1329, 12.5486) -> (59.0329, 10.6486) centre (59.0329, 12.5486) ccw
  line L72 (57.1329, 12.5486) -> (57.1329, 22.185)
  line L73 (59.0329, 24.085) -> (64.58, 24.085)
  line L74 (71.42, 24.085) -> (76.9671, 24.085)
  line L75 (78.8671, 22.185) -> (78.8671, 12.5486)
  line L76 (76.9671, 10.6486) -> (71.42, 10.6486)
  line L77 (59.0329, 10.6486) -> (64.58, 10.6486)
  arc A88 (53.1332, 17.0003) -> (54.1332, 18.0003) centre (53.1332, 18.0003) ccw
  arc A89 (54.375, 21.3462) -> (54.1332, 20.3929) centre (56.1332, 20.3929) ccw
  arc A90 (50.4658, 18.2968) -> (52.338, 17.0003) centre (52.338, 19.0003) ccw
  arc A91 (48.8669, 22.5339) -> (49.0486, 21.701) centre (50.8669, 22.5339) ccw
  arc A92 (57.547, 27.1966) -> (57.6108, 28.6871) centre (56.0518, 28.0073) ccw
  arc A93 (50.3863, 40.8048) -> (48.8662, 40.2807) centre (49.7166, 40.2807) ccw
  arc A94 (57.6108, 28.6871) -> (50.3863, 40.8048) centre (6.3199, 6.3202) ccw
  line L78 (53.1332, 17.0003) -> (52.338, 17.0003)
  line L79 (50.4658, 18.2968) -> (49.0486, 21.701)
  line L80 (48.8669, 22.5339) -> (48.8662, 40.2807)
  line L81 (57.547, 27.1966) -> (54.375, 21.3462)
  line L82 (54.1332, 20.3929) -> (54.1332, 18.0003)
  arc A95 (81.8674, 18.0003) -> (82.8674, 17.0003) centre (82.8674, 18.0003) ccw
  arc A96 (83.6626, 17.0003) -> (85.5348, 18.2968) centre (83.6626, 19.0003) ccw
  arc A97 (81.8674, 20.3929) -> (81.6256, 21.3462) centre (79.8674, 20.3929) ccw
  arc A98 (86.952, 21.701) -> (87.1337, 22.5339) centre (85.1337, 22.5339) ccw
  arc A99 (87.1344, 40.2807) -> (85.6143, 40.8048) centre (86.284, 40.2807) ccw
  line L83 (87.1337, 22.5339) -> (87.1344, 40.2807)
  line L84 (86.952, 21.701) -> (85.5348, 18.2968)
  line L85 (81.8674, 18.0003) -> (81.8674, 20.3929)
  arc A100 (58.596, 30.5755) -> (59.3603, 30.5411) centre (58.9865, 30.7437) ccw
  arc A101 (50.7936, 44.7904) -> (50.3034, 44.1264) centre (50.6309, 44.3976) ccw
  arc A102 (58.596, 30.5755) -> (50.3034, 44.1264) centre (7.2052, 8.4392) ccw
  line L86 (61.918, 40.1825) -> (50.7936, 44.7904)
  arc A103 (76.6397, 30.5411) -> (77.404, 30.5755) centre (77.0135, 30.7437) ccw
  arc A104 (74.082, 40.1825) -> (73.0266, 37.2051) centre (74.8956, 38.2184) ccw
  arc A105 (85.6966, 44.1264) -> (85.2064, 44.7904) centre (85.3691, 44.3976) ccw
  arc A106 (85.6966, 44.1264) -> (77.404, 30.5755) centre (128.7948, 8.4392) ccw
  line L87 (76.6397, 30.5411) -> (73.0266, 37.2051)
  line L88 (74.082, 40.1825) -> (85.2064, 44.7904)
  arc A107 (89.6849, 28.1023) -> (91.2524, 27.6451) centre (90.5353, 28.1023) ccw
  arc A108 (108.3552, 44.7479) -> (107.898, 46.3154) centre (107.898, 45.465) ccw
  arc A109 (91.8109, 46.3154) -> (89.6849, 44.1894) centre (91.8109, 44.1894) ccw
  line L89 (91.8109, 46.3154) -> (107.898, 46.3154)
  line L90 (89.6849, 44.1894) -> (89.6849, 28.1023)
  arc A110 (108.3552, 44.7479) -> (91.2524, 27.6451) centre (138.445, -2.4447) ccw
  arc A111 (64.7316, 4.7048) -> (61.3754, 5.9986) centre (61.3754, 0.9986) ccw
  line L91 (61.3754, 5.9986) -> (61.0697, 5.9986)
  line L92 (83.6626, 17.0003) -> (82.8674, 17.0003)
  arc A112 (123.4514, 57.1329) -> (125.3514, 59.0329) centre (123.4514, 59.0329) ccw
  arc A113 (111.915, 59.0329) -> (113.815, 57.1329) centre (113.815, 59.0329) ccw
  arc A114 (125.3514, 71.42) -> (125.3514, 64.58) centre (128.8174, 68) ccw
  arc A115 (111.915, 64.58) -> (111.915, 71.42) centre (108.495, 68) ccw
  arc A116 (113.815, 78.8671) -> (111.915, 76.9671) centre (113.815, 76.9671) ccw
  arc A117 (125.3514, 76.9671) -> (123.4514, 78.8671) centre (123.4514, 76.9671) ccw
  line L93 (125.3514, 64.58) -> (125.3514, 59.0329)
  line L94 (123.4514, 57.1329) -> (113.815, 57.1329)
  line L95 (111.915, 59.0329) -> (111.915, 64.58)
  line L96 (111.915, 71.42) -> (111.915, 76.9671)
  line L97 (125.3514, 71.42) -> (125.3514, 76.9671)
  line L98 (123.4514, 78.8671) -> (113.815, 78.8671)
  arc A118 (102.906, 64.2927) -> (104.2575, 65.6561) centre (103.3826, 65.1718) ccw
  arc A119 (104.2575, 70.3445) -> (102.906, 71.7079) centre (103.3826, 70.8288) ccw
  arc A120 (97.6891, 68.8794) -> (97.6891, 67.1212) centre (98.1657, 68.0003) ccw
  line L99 (97.6891, 67.1212) -> (102.906, 64.2927)
  line L100 (97.6891, 68.8794) -> (102.906, 71.7079)
  arc A121 (119, 53.1329) -> (118, 54.1329) centre (118, 53.1329) ccw
  arc A122 (117.7035, 50.4655) -> (119, 52.3377) centre (117, 52.3377) ccw
  arc A123 (113.4665, 48.8666) -> (114.2993, 49.0483) centre (113.4664, 50.8666) ccw
  arc A124 (95.1955, 50.386) -> (95.7196, 48.8659) centre (95.7196, 49.7163) ccw
  arc A125 (108.8037, 57.5467) -> (107.3132, 57.6105) centre (107.993, 56.0515) ccw
  arc A126 (114.6541, 54.3747) -> (115.6074, 54.1329) centre (115.6074, 56.1329) ccw
  arc A127 (107.3132, 57.6105) -> (95.1955, 50.386) centre (129.6801, 6.3196) ccw
  arc A128 (117.7035, 50.4655) -> (114.2993, 49.0483) centre (136.1983, 1.2434) ccw
  line L101 (115.6074, 54.1329) -> (118, 54.1329)
  line L102 (119, 52.3377) -> (119, 53.1329)
  line L103 (114.6541, 54.3747) -> (108.8037, 57.5467)
  line L104 (113.4665, 48.8666) -> (95.7196, 48.8659)
  arc A129 (104.2575, 70.3445) -> (104.2575, 65.6561) centre (108.4919, 68.0003) ccw
  arc A130 (64.2924, 33.0943) -> (65.6558, 31.7428) centre (65.1715, 32.6177) ccw
  arc A131 (68.8791, 38.3112) -> (67.1209, 38.3112) centre (68, 37.8346) ccw
  line L105 (68.8791, 38.3112) -> (71.7076, 33.0943)
  line L106 (64.2924, 33.0943) -> (67.1209, 38.3112)
  arc A132 (70.3442, 31.7428) -> (71.7076, 33.0943) centre (70.8285, 32.6177) ccw
  arc A133 (70.3442, 31.7428) -> (65.6558, 31.7428) centre (68, 27.5084) ccw
  line L107 (62.9734, 37.2051) -> (59.3603, 30.5411)
  arc A134 (62.9734, 37.2051) -> (61.918, 40.1825) centre (61.1044, 38.2184) ccw
  line L108 (78.4536, 27.1966) -> (81.6256, 21.3462)
  arc A135 (78.3898, 28.6871) -> (78.4536, 27.1966) centre (79.9488, 28.0073) ccw
  arc A136 (85.6143, 40.8048) -> (78.3898, 28.6871) centre (129.6807, 6.3202) ccw
  arc A137 (30.5408, 59.3606) -> (30.5752, 58.5963) centre (30.7434, 58.9868) ccw
  line L109 (30.5408, 59.3606) -> (37.2048, 62.9737)
  arc A138 (28.6868, 57.6105) -> (27.1963, 57.5467) centre (28.007, 56.0515) ccw
  line L110 (27.1963, 57.5467) -> (21.3459, 54.3747)
  arc A139 (40.8045, 50.386) -> (28.6868, 57.6105) centre (6.3199, 6.3196) ccw
  arc A140 (21.3459, 81.6253) -> (20.3926, 81.8671) centre (20.3926, 79.8671) ccw
  line L111 (20.3926, 81.8671) -> (18, 81.8671)
  arc A141 (5.9986, 74.9303) -> (4.5341, 78.4659) centre (0.9986, 74.9303) ccw
  arc A142 (4.7048, 71.2684) -> (5.9986, 74.6246) centre (0.9986, 74.6246) ccw
  line L112 (5.9986, 74.6246) -> (5.9986, 74.9303)
  line L113 (4.5341, 78.4659) -> (0.2929, 82.7071)
  arc A143 (50.1297, 0.9388) -> (51.1278, 0) centre (51.1278, 1) ccw
  arc A144 (52.5858, 0) -> (53.2929, 0.2929) centre (52.5858, 1) ccw
  line L114 (52.5858, 0) -> (51.1278, 0)
  line L115 (53.2929, 0.2929) -> (57.5341, 4.5341)
  arc A145 (91.2099, 50.7939) -> (91.8739, 50.3037) centre (91.6027, 50.6312) ccw
  arc A146 (98.7952, 62.9737) -> (95.8178, 61.9183) centre (97.7819, 61.1047) ccw
  arc A147 (105.4248, 58.5963) -> (105.4592, 59.3606) centre (105.2566, 58.9868) ccw
  line L116 (105.4592, 59.3606) -> (98.7952, 62.9737)
  line L117 (95.8178, 61.9183) -> (91.2099, 50.7939)
  arc A148 (105.4248, 58.5963) -> (91.8739, 50.3037) centre (127.5611, 7.2055) ccw
  arc A149 (105.4592, 76.64) -> (105.4248, 77.4043) centre (105.2566, 77.0138) ccw
  arc A150 (95.8178, 74.0823) -> (98.7952, 73.0269) centre (97.7819, 74.8959) ccw
  arc A151 (91.8739, 85.6969) -> (91.2099, 85.2067) centre (91.6027, 85.3694) ccw
  line L118 (98.7952, 73.0269) -> (105.4592, 76.64)
  line L119 (95.8178, 74.0823) -> (91.2099, 85.2067)
  arc A152 (91.8739, 85.6969) -> (105.4248, 77.4043) centre (127.5611, 128.7951) ccw
  arc A153 (118, 81.8671) -> (119, 82.8671) centre (118, 82.8671) ccw
  arc A154 (119, 83.6623) -> (117.7035, 85.5345) centre (117, 83.6623) ccw
  arc A155 (115.6074, 81.8671) -> (114.6541, 81.6253) centre (115.6074, 79.8671) ccw
  arc A156 (114.2993, 86.9517) -> (113.4665, 87.1334) centre (113.4664, 85.1334) ccw
  arc A157 (107.3132, 78.3895) -> (108.8037, 78.4533) centre (107.993, 79.9485) ccw
  arc A158 (95.7196, 87.1341) -> (95.1955, 85.614) centre (95.7196, 86.2837) ccw
  line L120 (95.7196, 87.1341) -> (113.4665, 87.1334)
  line L121 (119, 83.6623) -> (119, 82.8671)
  line L122 (115.6074, 81.8671) -> (118, 81.8671)
  line L123 (114.6541, 81.6253) -> (108.8037, 78.4533)
  arc A159 (114.2993, 86.9517) -> (117.7035, 85.5345) centre (136.1983, 134.7566) ccw
  arc A160 (95.1955, 85.614) -> (107.3132, 78.3895) centre (129.6801, 129.6804) ccw
  arc A161 (107.898, 89.6852) -> (108.3552, 91.2527) centre (107.898, 90.5356) ccw
  arc A162 (89.6849, 91.8112) -> (91.8109, 89.6852) centre (91.8109, 91.8112) ccw
  arc A163 (91.2524, 108.3555) -> (89.6849, 107.8983) centre (90.5353, 107.8983) ccw
  line L124 (89.6849, 91.8112) -> (89.6849, 107.8983)
  line L125 (91.8109, 89.6852) -> (107.898, 89.6852)
  arc A164 (91.2524, 108.3555) -> (108.3552, 91.2527) centre (138.445, 138.4453) ccw
  arc A165 (71.42, 111.915) -> (64.58, 111.915) centre (68, 108.495) ccw
  arc A166 (76.9671, 111.915) -> (78.8671, 113.815) centre (76.9671, 113.815) ccw
  arc A167 (57.1329, 113.815) -> (59.0329, 111.915) centre (59.0329, 113.815) ccw
  arc A168 (59.0329, 125.3514) -> (57.1329, 123.4514) centre (59.0329, 123.4514) ccw
  arc A169 (78.8671, 123.4514) -> (76.9671, 125.3514) centre (76.9671, 123.4514) ccw
  arc A170 (64.58, 125.3514) -> (71.42, 125.3514) centre (68, 128.8174) ccw
  line L126 (71.42, 125.3514) -> (76.9671, 125.3514)
  line L127 (64.58, 125.3514) -> (59.0329, 125.3514)
  line L128 (78.8671, 113.815) -> (78.8671, 123.4514)
  line L129 (57.1329, 123.4514) -> (57.1329, 113.815)
  line L130 (59.0329, 111.915) -> (64.58, 111.915)
  line L131 (71.42, 111.915) -> (76.9671, 111.915)
  arc A171 (67.1209, 97.6888) -> (68.8791, 97.6888) centre (68, 98.1654) ccw
  arc A172 (61.918, 95.8181) -> (62.9734, 98.7955) centre (61.1044, 97.7822) ccw
  arc A173 (59.3603, 105.4595) -> (58.596, 105.4251) centre (58.9865, 105.2569) ccw
  arc A174 (50.3034, 91.8742) -> (50.7936, 91.2102) centre (50.6309, 91.603) ccw
  line L132 (50.7936, 91.2102) -> (61.918, 95.8181)
  line L133 (62.9734, 98.7955) -> (59.3603, 105.4595)
  arc A175 (50.3034, 91.8742) -> (58.596, 105.4251) centre (7.2052, 127.5614) ccw
  arc A176 (85.2064, 91.2102) -> (85.6966, 91.8742) centre (85.3691, 91.603) ccw
  arc A177 (73.0266, 98.7955) -> (74.082, 95.8181) centre (74.8956, 97.7822) ccw
  arc A178 (77.404, 105.4251) -> (76.6397, 105.4595) centre (77.0135, 105.2569) ccw
  line L134 (74.082, 95.8181) -> (85.2064, 91.2102)
  line L135 (73.0266, 98.7955) -> (76.6397, 105.4595)
  arc A179 (77.404, 105.4251) -> (85.6966, 91.8742) centre (128.7948, 127.5614) ccw
  arc A180 (82.8674, 119.0003) -> (81.8674, 118.0003) centre (82.8674, 118.0003) ccw
  arc A181 (85.5348, 117.7038) -> (83.6626, 119.0003) centre (83.6626, 117.0003) ccw
  arc A182 (87.1337, 113.4668) -> (86.952, 114.2996) centre (85.1337, 113.4667) ccw
  arc A183 (78.4536, 108.804) -> (78.3898, 107.3135) centre (79.9488, 107.9933) ccw
  arc A184 (81.6256, 114.6544) -> (81.8674, 115.6077) centre (79.8674, 115.6077) ccw
  arc A185 (85.6143, 95.1958) -> (87.1344, 95.7199) centre (86.284, 95.7199) ccw
  line L136 (87.1344, 95.7199) -> (87.1337, 113.4668)
  line L137 (83.6626, 119.0003) -> (82.8674, 119.0003)
  line L138 (81.8674, 118.0003) -> (81.8674, 115.6077)
  arc A186 (85.5348, 117.7038) -> (86.952, 114.2996) centre (134.7569, 136.1986) ccw
  arc A187 (78.3898, 107.3135) -> (85.6143, 95.1958) centre (129.6807, 129.6804) ccw
  line L139 (78.4536, 108.804) -> (81.6256, 114.6544)
  arc A188 (48.8662, 95.7199) -> (50.3863, 95.1958) centre (49.7166, 95.7199) ccw
  arc A189 (49.0486, 114.2996) -> (48.8669, 113.4668) centre (50.8669, 113.4667) ccw
  arc A190 (54.1332, 115.6683) -> (54.3742, 114.654) centre (56.1332, 115.6077) ccw
  arc A191 (54.1332, 118.0003) -> (53.1332, 119.0003) centre (53.1332, 118.0003) ccw
  arc A192 (52.338, 119.0003) -> (50.4658, 117.7038) centre (52.338, 117.0003) ccw
  arc A193 (57.6108, 107.3135) -> (57.547, 108.804) centre (56.0518, 107.9933) ccw
  line L140 (54.3742, 114.654) -> (57.547, 108.804)
  line L141 (53.1332, 119.0003) -> (52.338, 119.0003)
  line L142 (54.1332, 118.0003) -> (54.1332, 115.6683)
  line L143 (48.8662, 95.7199) -> (48.8669, 113.4668)
  arc A194 (49.0486, 114.2996) -> (50.4658, 117.7038) centre (1.2437, 136.1986) ccw
  arc A195 (50.3863, 95.1958) -> (57.6108, 107.3135) centre (6.3199, 129.6804) ccw
  arc A196 (71.7076, 102.9057) -> (70.3442, 104.2572) centre (70.8285, 103.3823) ccw
  arc A197 (65.6558, 104.2572) -> (64.2924, 102.9057) centre (65.1715, 103.3823) ccw
  arc A198 (65.6558, 104.2572) -> (70.3442, 104.2572) centre (68, 108.4916) ccw
  line L144 (67.1209, 97.6888) -> (64.2924, 102.9057)
  line L145 (71.7076, 102.9057) -> (68.8791, 97.6888)
  arc A199 (50.1297, 0.9388) -> (0.939, 50.1217) centre (-2.2631, -2.2716) ccw
  arc A200 (50.1297, 0.9388) -> (51.1278, 0) centre (51.1278, 1) ccw
  arc A201 (0, 51.1198) -> (0.939, 50.1217) centre (1, 51.1198) ccw
  line L146 (5.9986, 74.9303) -> (5.9986, 74.6246)
  arc A202 (5.9986, 74.9303) -> (4.5341, 78.4659) centre (0.9986, 74.9303) ccw
  arc A203 (0.9376, 85.8703) -> (50.1218, 135.0623) centre (-2.3433, 138.3348) ccw
  arc A204 (0.9376, 85.8703) -> (0, 84.8722) centre (1, 84.8722) ccw
  arc A205 (51.1198, 136) -> (50.1218, 135.0623) centre (51.1198, 135) ccw
  arc A206 (135.0596, 50.1296) -> (85.8784, 0.9406) centre (138.1819, -2.1735) ccw
  arc A207 (84.8801, 0) -> (85.8784, 0.9406) centre (84.8801, 1) ccw
  arc A208 (135.0596, 50.1296) -> (136, 51.1278) centre (135, 51.1278) ccw
  arc A209 (85.8703, 135.0624) -> (135.0622, 85.8782) centre (138.334, 138.3425) ccw
  arc A210 (85.8703, 135.0624) -> (84.8722, 136) centre (84.8722, 135) ccw
  arc A211 (136, 84.8802) -> (135.0622, 85.8782) centre (135, 84.8802) ccw
  circle A212 centre (27.5084, 68) radius 2.1
  circle A213 centre (108.4916, 68) radius 2.1
  circle A214 centre (68, 108.4916) radius 2.1
  circle A215 centre (68, 27.5084) radius 2.1
  line L147 (14, 83) -> (9, 83)
  line L148 (14, 53) -> (9, 53)
  line L149 (9, 83) -> (9, 85.1)
  line L150 (9, 85.1) -> (14, 85.1)
  line L151 (14, 85.1) -> (14, 83)
  line L152 (14, 53) -> (14, 50.9)
  line L153 (14, 50.9) -> (9, 50.9)
  line L154 (9, 50.9) -> (9, 53)
  line L155 (122, 83) -> (127, 83)
  line L156 (122, 53) -> (127, 53)
  line L157 (127, 83) -> (127, 85.1)
  line L158 (127, 85.1) -> (122, 85.1)
  line L159 (122, 85.1) -> (122, 83)
  line L160 (122, 53) -> (122, 50.9)
  line L161 (122, 50.9) -> (127, 50.9)
  line L162 (127, 50.9) -> (127, 53)
  line L163 (53, 122) -> (53, 127)
  line L164 (83, 122) -> (83, 127)
  line L165 (53, 127) -> (50.9, 127)
  line L166 (50.9, 127) -> (50.9, 122)
  line L167 (50.9, 122) -> (53, 122)
  line L168 (83, 122) -> (85.1, 122)
  line L169 (85.1, 122) -> (85.1, 127)
  line L170 (85.1, 127) -> (83, 127)
  line L171 (53, 14) -> (53, 9)
  line L172 (83, 14) -> (83, 9)
  line L173 (53, 9) -> (50.9, 9)
  line L174 (50.9, 9) -> (50.9, 14)
  line L175 (50.9, 14) -> (53, 14)
  line L176 (83, 14) -> (85.1, 14)
  line L177 (85.1, 14) -> (85.1, 9)
  line L178 (85.1, 9) -> (83, 9)
  line L179 (12.5486, 78.8671) -> (22.185, 78.8671)
  arc A216 (12.5486, 78.8671) -> (10.6486, 76.9671) centre (12.5486, 76.9671) ccw
  line L180 (10.6486, 76.9671) -> (10.6486, 71.42)
  line L181 (24.085, 71.42) -> (24.085, 76.9671)
  arc A217 (24.085, 76.9671) -> (22.185, 78.8671) centre (22.185, 76.9671) ccw
  line L182 (12.5486, 57.1329) -> (22.185, 57.1329)
  arc A218 (10.6486, 59.0329) -> (12.5486, 57.1329) centre (12.5486, 59.0329) ccw
  line L183 (10.6486, 59.0329) -> (10.6486, 64.58)
  line L184 (24.085, 64.58) -> (24.085, 59.0329)
  arc A219 (22.185, 57.1329) -> (24.085, 59.0329) centre (22.185, 59.0329) ccw
  arc A220 (10.6486, 64.58) -> (10.6486, 71.42) centre (7.1826, 68) ccw
  arc A221 (24.085, 71.42) -> (24.085, 64.58) centre (27.505, 68) ccw
  line L185 (123.4514, 78.8671) -> (113.815, 78.8671)
  arc A222 (125.3514, 76.9671) -> (123.4514, 78.8671) centre (123.4514, 76.9671) ccw
  line L186 (125.3514, 76.9671) -> (125.3514, 71.42)
  line L187 (111.915, 71.42) -> (111.915, 76.9671)
  arc A223 (113.815, 78.8671) -> (111.915, 76.9671) centre (113.815, 76.9671) ccw
  line L188 (123.4514, 57.1329) -> (113.815, 57.1329)
  arc A224 (123.4514, 57.1329) -> (125.3514, 59.0329) centre (123.4514, 59.0329) ccw
  line L189 (125.3514, 59.0329) -> (125.3514, 64.58)
  line L190 (111.915, 64.58) -> (111.915, 59.0329)
  arc A225 (111.915, 59.0329) -> (113.815, 57.1329) centre (113.815, 59.0329) ccw
  arc A226 (125.3514, 71.42) -> (125.3514, 64.58) centre (128.8174, 68) ccw
  arc A227 (111.915, 64.58) -> (111.915, 71.42) centre (108.495, 68) ccw
  line L191 (57.1329, 123.4514) -> (57.1329, 113.815)
  arc A228 (59.0329, 125.3514) -> (57.1329, 123.4514) centre (59.0329, 123.4514) ccw
  line L192 (59.0329, 125.3514) -> (64.58, 125.3514)
  line L193 (64.58, 111.915) -> (59.0329, 111.915)